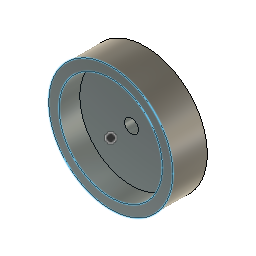
bouchon_loquet_placard_wc v2 (Autodesk Fusion 360 design; units mm, degrees)
Autodesk Fusion 360 part; units mm, degrees
sketch "Esquisse1" plane through (0, 0, 0) normal (0, 1, 0) x (1, 0, 0)
  circle A0 centre (0, 0) radius 9
  circle A1 centre (0, 0) radius 7.5
  dimension "d1" = 18
  dimension "d6" = 15
  constraint coincident A0.centre A1.centre
  measures "d1" diameter of A0
  measures "d6" diameter of A1
extrude "Extrusion2" add sketch "Esquisse1" along normal blind 5 contours A0 | A1
extrude "Extrusion3" cut sketch "Esquisse1" along normal blind 3 contours A1
sketch "Esquisse2" plane through (0, 5, 0) normal (0, 1, 0) x (-1, 0, 0)
  circle A0 centre (0, 0) radius 9
  circle A1 centre (0, 0) radius 1
  dimension "d9" = 2
  constraint coincident A0.centre A1.centre
  measures "d9" diameter of A1
extrude "Extrusion4" cut sketch "Esquisse2" against normal blind 3 contours A1
